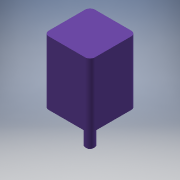
# Autodesk Inventor part: Nema 8
Saved by Autodesk Inventor 2016 (Build 200138000, 138)
## iProperties
Created: 2015-07-20
Part Number: Nema 8
Material: Generic
Document SubType Name: Modeling
Designer: bastli
Density: 1 g/cm^3
Appearance: Violet
Author: bastli
Autodesk Inventor part; units mm, degrees
ref_plane "YZ Plane" through (0, 0, 0) normal (1, 0, 0) x (0, 1, 0)
ref_plane "XZ Plane" through (0, 0, 0) normal (0, 1, 0) x (-1, 0, 0)
ref_plane "XY Plane" through (0, 0, 0) normal (0, 0, 1) x (1, 0, 0)
sketch "Sketch1" plane through (0, 0, 0) normal (0, 0, 1) x (1, 0, 0)
  circle A0 centre (-54.61, 0) radius 11.5 construction
  circle A1 centre (-66.11, 11.5) radius 1.3 construction
  circle A2 centre (-43.11, 11.5) radius 1.3 construction
  circle A3 centre (-66.11, -11.5) radius 1.3 construction
  circle A4 centre (-43.11, -11.5) radius 1.3 construction
  line L0 (-64.77, 10.16) -> (-44.45, 10.16)
  line L1 (-44.45, 10.16) -> (-44.45, -10.16)
  line L2 (-44.45, -10.16) -> (-64.77, -10.16)
  line L3 (-64.77, -10.16) -> (-64.77, 10.16)
  line L4 (-64.77, 10.16) -> (-44.45, -10.16) construction
  line L5 (-44.45, 10.16) -> (-64.77, -10.16) construction
  circle A5 centre (-54.61, 0) radius 7.495
  point P0 (0, 0)
  dimension "d0" = 20.32
  dimension "d1" = 20.32
  dimension "d2" = 14.99
  constraints: 12 end point, 5 coincident, 2 midpoint, 2 parallel, 1 centre point, 1 horizontal, 1 perpendicular
  measures "d0" distance of L0.start L0.end
  measures "d1" distance of L2.end L0.start
  measures "d2" diameter of A5
extrude "Extrusion1" add sketch "Sketch1" along normal blind 28 contours L0 L1 L2 L3 | A5
sketch "Sketch2" plane through (0, 0, 0) normal (0, 0, -1) x (-1, 0, 0)
  point P0 (0, 0)
  point P1 (66.11, -11.5)
  point P2 (43.11, -11.5)
  point P3 (43.11, 11.5)
  point P4 (66.11, 11.5)
hole "Hole1" at (-66.11, -11.5, 0) at (-43.11, -11.5, 0) at (-43.11, 11.5, 0) at (-66.11, 11.5, 0) direction (0, 0, 1) diameter 3 depth 8 tip angle 118
sketch "Sketch3" plane through (0, 0, 0) normal (0, 0, -1) x (-1, 0, 0)
  circle A0 centre (54.61, 0) radius 7.495 projected
  circle A1 centre (54.61, 0) radius 2
  point P0 (0, 0)
  dimension "d14" = 4
  constraints: 1 centre point, 1 coincident
  measures "d14" diameter of A1
extrude "Extrusion2" add sketch "Sketch3" along normal blind 1.5 contours A0 | A1
extrude "Extrusion3" add sketch "Sketch3" along normal blind 15 contours A1
chamfer "Chamfer1" distance 0.6 angle 45 1 edges at (-52.61, 0, -15)
fillet "Fillet1" radius 2.16 4 edges at (-64.77, -10.16, 14) (-64.77, 10.16, 14) (-44.45, -10.16, 14) (-44.45, 10.16, 14)
body "Solid1"
